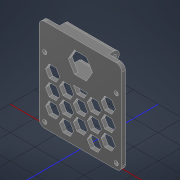
# Autodesk Inventor part: Base-Plate
Saved by Autodesk Inventor 2022.2 (Build 262287010, 287A)
## iProperties
Created: 2022-03-22
Part Number: Base-Plate
Material: ABS-Kunststoff
Document SubType Name: Modeling
Designer: sleib
Density: 1.06 g/cm^3
Appearance: Glatt - Schwarz
Author: sleib
Autodesk Inventor part; units mm, degrees
ref_plane "YZ Plane" through (0, 0, 0) normal (1, 0, 0) x (0, 1, 0)
ref_plane "XZ Plane" through (0, 0, 0) normal (0, 1, 0) x (-1, 0, 0)
ref_plane "XY Plane" through (0, 0, 0) normal (0, 0, 1) x (1, 0, 0)
sketch "Skizze1" plane through (0, 0, 0) normal (1, 0, 0) x (0, 1, 0)
  line L0 (33, 3) -> (-42, 3)
  line L1 (-42, 3) -> (-42, 0)
  line L2 (-42, 0) -> (33, 0)
  line L3 (33, 0) -> (33, 3)
  line L4 (33, 0) -> (25, 0)
  line L5 (25, 0) -> (25, -4.5)
  line L6 (25, -4.5) -> (33, -4.5) construction
  line L7 (33, -4.5) -> (33, 0)
  circle A0 centre (29, -4.5) radius 4
  line L8 (8, 0) -> (0, 0)
  line L9 (0, 0) -> (0, -8.5)
  line L10 (0, -8.5) -> (8, -8.5) construction
  line L11 (8, -8.5) -> (8, 0)
  circle A1 centre (4, -8.5) radius 4
  circle A2 centre (29, -4.5) radius 1.7
  circle A3 centre (4, -8.5) radius 1.7
  dimension "d0" = 75
  dimension "d1" = 3
  dimension "d2" = 8
  dimension "d5" = 4.5
  dimension "d6" = 8
  dimension "d7" = 8.5
  dimension "d8" = 25
  dimension "d9" = 3.4
  dimension "d10" = 3.4
  constraints: 24 end point, 6 parallel, 3 coincident, 3 horizontal, 3 perpendicular, 2 centre point, 2 midpoint, 1 point on line, 6 other
  measures "d0" distance between parallel lines of L1 L3
  measures "d1" distance of L2.end L0.start
  measures "d2" distance of L6.end L5.end
  measures "d5" distance between parallel lines of L4 L6
  measures "d6" distance of L10.end L9.end
  measures "d7" distance between parallel lines of L10 L8
  measures "d8" horizontal distance of point (4, -8.5) point (29, -4.5)
  measures "d9" diameter of A2
  measures "d10" diameter of A3
extrude "Extrusion1" add sketch "Skizze1" along normal mid plane 67 contours L3 L2 L1 L0
extrude "Extrusion2" add sketch "Skizze1" along normal mid plane 40 contours L7 A0 L5 L2 | A0
extrude "Extrusion3" add sketch "Skizze1" along normal mid plane 26 contours L2 L11 A1 L9 | A1
sketch "Skizze3" plane through (33.5, -42, 0) normal (0, 0, -1) x (-1, 0, 0)
  line L0 (46.5, 50) -> (46.5, 42) projected
  line L1 (46.5, 42) -> (20.5, 42) projected
  line L2 (20.5, 42) -> (20.5, 50) projected
  line L3 (20.5, 50) -> (46.5, 50) projected
  line L4 (13.5, 67) -> (13.5, 75) projected
  line L5 (13.5, 75) -> (0, 75) projected
  line L6 (0, 0) -> (0, 75) projected
  line L7 (0, 0) -> (67, 0) projected
  line L8 (67, 75) -> (67, 0) projected
  line L9 (67, 75) -> (53.5, 75) projected
  line L10 (53.5, 75) -> (53.5, 67) projected
  line L11 (53.5, 67) -> (13.5, 67) projected
  circle A0 centre (4.5, 4.5) radius 4.5 construction
  circle A1 centre (62.5, 4.5) radius 4.5 construction
  line L12 (0, 0) -> (0, 75) projected
  line L13 (67, 75) -> (67, 0) projected
  line L14 (0, 0) -> (67, 0) projected
  circle A2 centre (4.5, 4.5) radius 1.7
  circle A3 centre (62.5, 4.5) radius 1.7
  circle A4 centre (4.5, 53.5) radius 1.7
  circle A5 centre (62.5, 53.5) radius 1.7
  line L15 (67, 75) -> (0, 75) construction
  line L16 (33.5, 75) -> (33.5, 0) construction
  line L17 (67, 0) -> (0, 0) construction
  line L18 (38.4075, 50) -> (28.5925, 50)
  line L19 (28.5925, 50) -> (23.685, 58.5)
  line L20 (23.685, 58.5) -> (28.5925, 67)
  line L21 (28.5925, 67) -> (38.4075, 67)
  line L22 (38.4075, 67) -> (43.315, 58.5)
  line L23 (43.315, 58.5) -> (38.4075, 50)
  line L24 (53.5, 67) -> (13.5, 67) projected
  line L25 (46.5, 50) -> (20.5, 50) projected
  circle A6 centre (4.5, 4.5) radius 3
  circle A7 centre (62.5, 4.5) radius 3
  circle A8 centre (62.5, 53.5) radius 3
  circle A9 centre (4.5, 53.5) radius 3
  line L26 (13.8701, 37) -> (8.0966, 37)
  line L27 (8.0966, 37) -> (5.2098, 42)
  line L28 (5.2098, 42) -> (8.0966, 47)
  line L29 (8.0966, 47) -> (13.8701, 47)
  line L30 (13.8701, 47) -> (16.7568, 42)
  line L31 (16.7568, 42) -> (13.8701, 37)
  line L32 (25.1284, 30.5) -> (19.3549, 30.5)
  line L33 (19.3549, 30.5) -> (16.4682, 35.5)
  line L34 (16.4682, 35.5) -> (19.3549, 40.5)
  line L35 (19.3549, 40.5) -> (25.1284, 40.5)
  line L36 (25.1284, 40.5) -> (28.0152, 35.5)
  line L37 (28.0152, 35.5) -> (25.1284, 30.5)
  line L38 (170.3307, 42) -> (-28.3884, 42) construction
  line L39 (33.5, -15) -> (33.5, 90) construction
  line L40 (30.6132, 37) -> (27.7265, 42)
  line L41 (27.7265, 42) -> (30.6132, 47)
  line L42 (30.6132, 47) -> (36.3868, 47)
  line L43 (36.3868, 37) -> (30.6132, 37)
  line L44 (36.3868, 47) -> (39.2735, 42)
  line L45 (39.2735, 42) -> (36.3868, 37)
  line L46 (53.1299, 37) -> (50.2432, 42)
  line L47 (50.2432, 42) -> (53.1299, 47)
  line L48 (53.1299, 47) -> (58.9034, 47)
  line L49 (58.9034, 37) -> (53.1299, 37)
  line L50 (58.9034, 47) -> (61.7902, 42)
  line L51 (61.7902, 42) -> (58.9034, 37)
  line L52 (8.0966, 24) -> (5.2098, 29)
  line L53 (5.2098, 29) -> (8.0966, 34)
  line L54 (8.0966, 34) -> (13.8701, 34)
  line L55 (13.8701, 24) -> (8.0966, 24)
  line L56 (13.8701, 34) -> (16.7568, 29)
  line L57 (16.7568, 29) -> (13.8701, 24)
  line L58 (30.6132, 24) -> (27.7265, 29)
  line L59 (27.7265, 29) -> (30.6132, 34)
  line L60 (30.6132, 34) -> (36.3868, 34)
  line L61 (36.3868, 24) -> (30.6132, 24)
  line L62 (36.3868, 34) -> (39.2735, 29)
  line L63 (39.2735, 29) -> (36.3868, 24)
  line L64 (53.1299, 24) -> (50.2432, 29)
  line L65 (50.2432, 29) -> (53.1299, 34)
  line L66 (53.1299, 34) -> (58.9034, 34)
  line L67 (58.9034, 24) -> (53.1299, 24)
  line L68 (58.9034, 34) -> (61.7902, 29)
  line L69 (61.7902, 29) -> (58.9034, 24)
  line L70 (8.0966, 11) -> (5.2098, 16)
  line L71 (5.2098, 16) -> (8.0966, 21)
  line L72 (8.0966, 21) -> (13.8701, 21)
  line L73 (13.8701, 11) -> (8.0966, 11)
  line L74 (13.8701, 21) -> (16.7568, 16)
  line L75 (16.7568, 16) -> (13.8701, 11)
  line L76 (30.6132, 11) -> (27.7265, 16)
  line L77 (27.7265, 16) -> (30.6132, 21)
  line L78 (30.6132, 21) -> (36.3868, 21)
  line L79 (36.3868, 11) -> (30.6132, 11)
  line L80 (36.3868, 21) -> (39.2735, 16)
  line L81 (39.2735, 16) -> (36.3868, 11)
  line L82 (53.1299, 11) -> (50.2432, 16)
  line L83 (50.2432, 16) -> (53.1299, 21)
  line L84 (53.1299, 21) -> (58.9034, 21)
  line L85 (58.9034, 11) -> (53.1299, 11)
  line L86 (58.9034, 21) -> (61.7902, 16)
  line L87 (61.7902, 16) -> (58.9034, 11)
  line L88 (38.9848, 35.5) -> (41.8716, 40.5)
  line L89 (41.8716, 30.5) -> (38.9848, 35.5)
  line L90 (41.8716, 40.5) -> (47.6451, 40.5)
  line L91 (47.6451, 30.5) -> (41.8716, 30.5)
  line L92 (47.6451, 40.5) -> (50.5318, 35.5)
  line L93 (50.5318, 35.5) -> (47.6451, 30.5)
  line L94 (16.4682, 22.5) -> (19.3549, 27.5)
  line L95 (19.3549, 17.5) -> (16.4682, 22.5)
  line L96 (19.3549, 27.5) -> (25.1284, 27.5)
  line L97 (25.1284, 17.5) -> (19.3549, 17.5)
  line L98 (25.1284, 27.5) -> (28.0152, 22.5)
  line L99 (28.0152, 22.5) -> (25.1284, 17.5)
  line L100 (38.9848, 22.5) -> (41.8716, 27.5)
  line L101 (41.8716, 17.5) -> (38.9848, 22.5)
  line L102 (41.8716, 27.5) -> (47.6451, 27.5)
  line L103 (47.6451, 17.5) -> (41.8716, 17.5)
  line L104 (47.6451, 27.5) -> (50.5318, 22.5)
  line L105 (50.5318, 22.5) -> (47.6451, 17.5)
  line L106 (16.4682, 9.5) -> (19.3549, 14.5)
  line L107 (19.3549, 4.5) -> (16.4682, 9.5)
  line L108 (19.3549, 14.5) -> (25.1284, 14.5)
  line L109 (25.1284, 4.5) -> (19.3549, 4.5)
  line L110 (25.1284, 14.5) -> (28.0152, 9.5)
  line L111 (28.0152, 9.5) -> (25.1284, 4.5)
  line L112 (38.9848, 9.5) -> (41.8716, 14.5)
  line L113 (41.8716, 4.5) -> (38.9848, 9.5)
  line L114 (41.8716, 14.5) -> (47.6451, 14.5)
  line L115 (47.6451, 4.5) -> (41.8716, 4.5)
  line L116 (47.6451, 14.5) -> (50.5318, 9.5)
  line L117 (50.5318, 9.5) -> (47.6451, 4.5)
  line L118 (46.5, 42) -> (20.5, 42) projected
  line L119 (27.7265, 42) -> (39.2735, 42)
  line L120 (46.5, 42) -> (20.5, 42) projected
  point P0 (33.5, 42)
  point P1 (33.5, 58.5)
  point P2 (10.9833, 42)
  point P3 (22.2417, 35.5)
  point P4 (33.5, 42)
  point P5 (56.0167, 42)
  point P6 (10.9833, 29)
  point P7 (33.5, 29)
  point P8 (56.0167, 29)
  point P9 (10.9833, 16)
  point P10 (33.5, 16)
  point P11 (56.0167, 16)
  point P12 (44.7583, 35.5)
  point P13 (22.2417, 22.5)
  point P14 (44.7583, 22.5)
  point P15 (22.2417, 9.5)
  point P16 (44.7583, 9.5)
  dimension "d19" = 9
  dimension "d20" = 3.4
  dimension "d21" = 49
  dimension "d25" = 6
  dimension "d28" = 10
  dimension "d29" = 10
  dimension "d30" = 3
  dimension "d31" = 1.5
  dimension "d32" = 11.2583
  dimension "d35" = 22.5167
  dimension "d38" = 13
  dimension "d43" = 22.5167
  dimension "d46" = 13
  constraints: 196 end point, 10 centre point, 7 equal radius, 6 coincident, 4 horizontal, 4 tangent, 3 collinear, 3 point on line, 2 midpoint, 2 vertical, 2 vertical alignment, 1 horizontal alignment, 208 other
  measures "d19" diameter of A0
  measures "d20" diameter of A2
  measures "d21" distance of A2.centre A4.centre
  measures "d25" diameter of A6
  measures "d28" distance between parallel lines of L26 L29
  measures "d29" distance between parallel lines of L32 L35
  measures "d30" distance between parallel lines of L34 L31
  measures "d31" distance from line of L35 L30.end
  measures "d32" horizontal distance of point (22.242, 35.5) point (10.983, 42)
  measures "d35" distance of L27.end L40.end
  measures "d38" distance of L27.end L52.end
  measures "d43" distance of L34.end L88.end
  measures "d46" distance of L34.end L94.end
extrude "Extrusion4" cut sketch "Skizze3" against normal through all contours L3 L19 L20 L11 L22 L23 | L45 L43 L40 L1 | A2 | A3 | A4 | A5 | L26 L27 L28 L29 L30 L31 | L32 L33 L34 L35 L36 L37 | L46 L47 L48 L50 L51 L49 | L52 L53 L54 L56 L57 L55 | L58 L59 L60 L62 L63 L61 | L64 L65 L66 L68 L69 L67 | L70 L71 L72 L74 L75 L73 | L76 L77 L78 L80 L81 L79 | L82 L83 L84 L86 L87 L85 | L88 L90 L92 L93 L91 L89 | L94 L96 L98 L99 L97 L95 | L100 L102 L104 L105 L103 L101 | L106 L108 L110 L111 L109 L107 | L112 L114 L116 L117 L115 L113
extrude "Extrusion5" cut sketch "Skizze3" against normal blind 1 contours A6 | A7 | A8 | A9
fillet "Rundung1" radius 4.5 4 edges at (33.5, -42, 1.5) (-33.5, -42, 1.5) (-33.5, 33, 1.5) (33.5, 33, 1.5)
equation "\"d29\" = d28"
equation "\"d31\" = 0.5 * d30"
equation "\"d35\" = 2 * d32"
equation "\"d38\" = d28 + d30"
equation "\"d43\" = 2 * d32"
equation "\"d46\" = d28 + d30"
